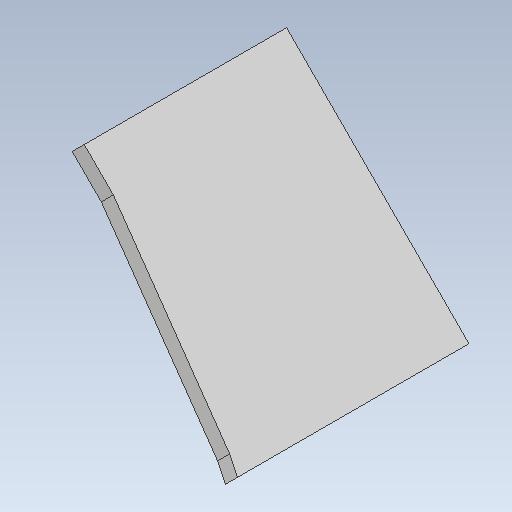
# Autodesk Inventor part: diagonal
Saved by Autodesk Inventor 2020 (Build 240168000, 168)
## iProperties
Created: 2020-04-24
Part Number: diagonal
Material: Genérico
Document SubType Name: Modeling
Designer: gi-se
Density: 1 g/cm^3
Appearance: Padrão
Author: gi-se
Autodesk Inventor part; units mm, degrees
ref_plane "YZ Plane" through (0, 0, 0) normal (1, 0, 0) x (0, 1, 0)
ref_plane "XZ Plane" through (0, 0, 0) normal (0, 1, 0) x (-1, 0, 0)
ref_plane "XY Plane" through (0, 0, 0) normal (0, 0, 1) x (1, 0, 0)
sketch "Esboço1" plane through (0, 0, 0) normal (0, 0, 1) x (1, 0, 0)
  line L0 (-71, -40) -> (-71, -37)
  line L1 (-71, -37) -> (-38.1386, -69.8614)
  line L2 (14.6, -69.1) -> (-41.9, -69.1) projected
  line L3 (-38.9, -69.1) -> (-71, -37)
  line L4 (-71, -37) -> (-73.1213, -39.1213)
  line L5 (-73.1213, -39.1213) -> (-41.0213, -71.2213)
  line L6 (-41.0213, -71.2213) -> (-38.9, -69.1)
  point P0 (0, 0)
  dimension "d0" = 3
  dimension "d1" = 45
  dimension "d2" = 3
  constraints: 12 end point, 2 parallel, 2 point on line, 1 collinear, 1 perpendicular, 1 vertical
  measures "d0" distance of L0.start L0.end
  measures "d1" angle of L0 L1
  measures "d2" distance of L4.end L0.end
extrude "Extrusão1" add sketch "Esboço1" against normal blind 11.5
sketch "Esboço3" plane through (0, 0, 0) normal (0, 0, 1) x (1, 0, 0)
  line L0 (-38.9, -69.1) -> (-41.0213, -71.2213) projected
  line L1 (-38.9, -69.1) -> (-71, -37)
  line L2 (-71, -37) -> (-73.1213, -39.1213)
  line L3 (-73.1213, -39.1213) -> (-41.0213, -71.2213)
  line L4 (-41.0213, -71.2213) -> (-38.9, -69.1)
  point P0 (0, 0)
  constraints: 8 end point, 2 parallel, 1 perpendicular
extrude "Extrusão2" add sketch "Esboço3" along normal blind 35.6
sketch "Esboço6" plane through (-73.1213, -39.1213, 35.6) normal (-0.7071, -0.7071, 0) x (-0.7071, 0.7071, 0)
  line L0 (-42.3963, 7.117) -> (-7.2426, 11.5) projected
  line L1 (55.3259, 11.5) -> (-7.2426, 11.5) projected
  line L2 (-42.3963, 7.117) -> (-83.2265, -3.0646) projected
  line L3 (-45.3963, 0) -> (0, 0) projected
  line L4 (-45.3963, 47.1) -> (-45.3963, 0) projected
  line L5 (0, 0) -> (-45.3963, 0)
  line L6 (-45.3963, 0) -> (-45.3963, 14)
  line L7 (-45.3963, 14) -> (0, 14)
  line L8 (0, 14) -> (0, 0)
  point P0 (-24.0416, 35.6)
  point P1 (-45.3963, 6.3689)
  point P2 (0, 11.5)
  constraints: 8 end point, 2 parallel, 1 horizontal, 1 perpendicular, 1 point on line
extrude "Extrusão3" cut sketch "Esboço6" against normal blind 19 contours L0 L1 L8 L3 L4 L2
